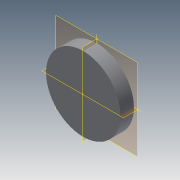
# Autodesk Inventor part: 101050-003
Saved by Autodesk Inventor 2015 SP1 (Build 190203100, 203)
## iProperties
Created: 2015-12-19
Part Number: 101050-003
Material: Generic
Document SubType Name: Modeling
Designer: Yamaura
Density: 1 g/cm^3
Appearance: Default
Author: Yamaura
Autodesk Inventor part; units mm, degrees
sketch "スケッチ1" plane through (0, 0, 0) normal (0, 0, 1) x (1, 0, 0)
  circle A0 centre (0, 0) radius 1.395
  dimension "d0" = 2.79
  constraints: 1 centre point, 1 coincident
  measures "d0" diameter of A0
extrude "押し出し1" add sketch "スケッチ1" along normal blind 0.51
